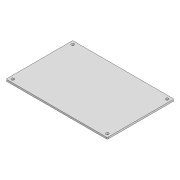
# Autodesk Inventor part: Base
Saved by Autodesk Inventor 2020 (Build 240168000, 168)
## iProperties
Created: 2022-07-16
Part Number: Base
Material: Genérico
Document SubType Name: Modeling
Designer: gabri
Density: 1 g/cm^3
Appearance: Padrão
Author: gabri
Autodesk Inventor part; units mm, degrees
ref_plane "YZ Plane" through (0, 0, 0) normal (1, 0, 0) x (0, 1, 0)
ref_plane "XZ Plane" through (0, 0, 0) normal (0, 1, 0) x (-1, 0, 0)
ref_plane "XY Plane" through (0, 0, 0) normal (0, 0, 1) x (1, 0, 0)
sketch "Esboço1" plane through (0, 0, 0) normal (0, 1, 0) x (-1, 0, 0)
  line L0 (0, 0) -> (240, 0)
  line L1 (240, 0) -> (240, -158)
  line L2 (240, -158) -> (0, -158)
  line L3 (0, -158) -> (0, 0)
  dimension "d0" = 240
  dimension "d1" = 158
  constraints: 8 end point, 2 parallel, 1 horizontal, 1 perpendicular
  measures "d0" distance of L1.end L2.end
  measures "d1" distance of L0.end L1.end
extrude "Extrusão1" add sketch "Esboço1" along normal blind 4
fillet "Arredondamento1" radius 2 4 edges at (0, 2, 0) (0, 2, -158) (-240, 2, 0) (-240, 2, -158)
sketch "Esboço2" plane through (0, 4, 0) normal (0, 1, 0) x (1, 0, 0)
  circle A0 centre (-232, 150) radius 3.35
  circle A1 centre (-232, 8) radius 3.35
  circle A2 centre (-8, 150) radius 3.35
  circle A3 centre (-8, 8) radius 3.35
  line L0 (-240, 156) -> (-240, 2) projected
  line L1 (-2, 158) -> (-238, 158) projected
  line L2 (-238, 0) -> (-2, 0) projected
  line L3 (0, 2) -> (0, 156) projected
  point P0 (0, 0)
  dimension "d5" = 6.7
  dimension "d6" = 6.7
  dimension "d7" = 6.7
  dimension "d8" = 6.7
  dimension "d9" = 8
  dimension "d10" = 8
  dimension "d11" = 8
  dimension "d12" = 8
  dimension "d13" = 8
  dimension "d14" = 8
  dimension "d15" = 8
  dimension "d16" = 8
  constraints: 4 centre point
  measures "d5" diameter of A1
  measures "d6" diameter of A2
  measures "d7" diameter of A3
  measures "d8" diameter of A0
  measures "d9" distance from line of L0 A0.centre
  measures "d10" distance from line of L1 A0.centre
  measures "d11" distance from line of L2 A1.centre
  measures "d12" distance from line of L0 A1.centre
  measures "d13" distance from line of L3 A3.centre
  measures "d14" distance from line of L2 A3.centre
  measures "d15" distance from line of L3 A2.centre
  measures "d16" distance from line of L1 A2.centre
extrude "Extrusão2" cut sketch "Esboço2" against normal blind 10
equation "\"d8\" = d6"
equation "\"d10\" = d12"
equation "\"d11\" = d10"
equation "\"d12\" = d9"
equation "\"d13\" = d12"
equation "\"d14\" = d13"
equation "\"d15\" = d13"
equation "\"d16\" = d15"
